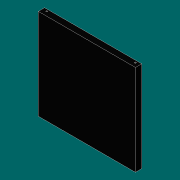
# Autodesk Inventor part: front
Saved by Autodesk Inventor 2016 SP1 (Build 200210100, 210)
## iProperties
Created: 2015-10-13
Part Number: front
Material: PC/ABS Plastic
Document SubType Name: Modeling
Designer: Sawaiz
Density: 0.357273 g/cm^3
Appearance: Smooth - Black
Author: Sawaiz
Autodesk Inventor part; units mm, degrees
ref_plane "YZ Plane" through (0, 0, 0) normal (1, 0, 0) x (0, 1, 0)
ref_plane "XZ Plane" through (0, 0, 0) normal (0, 1, 0) x (-1, 0, 0)
ref_plane "XY Plane" through (0, 0, 0) normal (0, 0, 1) x (1, 0, 0)
sketch "Sketch1" plane through (0, 0, 0) normal (1, 0, 0) x (0, 1, 0)
  line L0 (-73.025, -68.2625) -> (73.025, -68.2625)
  line L1 (73.025, -68.2625) -> (73.025, 68.2625)
  line L2 (73.025, 68.2625) -> (-73.025, 68.2625)
  line L3 (-73.025, 68.2625) -> (-73.025, -68.2625)
  line L4 (-73.025, -68.2625) -> (73.025, 68.2625) construction
  line L5 (73.025, -68.2625) -> (-73.025, 68.2625) construction
  point P0 (0, 0)
  dimension "d0" = 146.05
  dimension "d1" = 136.525
  constraints: 12 end point, 2 midpoint, 2 parallel, 1 horizontal, 1 perpendicular
  measures "d0" distance of L2.end L1.end
  measures "d1" distance of L1.end L0.end
extrude "Extrusion1" add sketch "Sketch1" along normal blind 9.525
sketch "Sketch5" plane through (0, -73.025, 68.2625) normal (0, 0, 1) x (1, 0, 0)
  line L0 (0, 146.05) -> (0, 0) projected
  line L1 (0, 0) -> (9.525, 0) projected
  line L2 (9.525, 146.05) -> (9.525, 0) projected
  line L3 (0, 146.05) -> (9.525, 146.05) projected
  line L4 (0, 146.05) -> (9.525, 146.05) projected
  line L5 (3.175, 146.05) -> (3.175, 0)
  point P0 (0, 73.025)
  point P1 (3.175, 139.7)
  point P2 (3.175, 6.35)
  dimension "d35" = 6.35
  dimension "d36" = 6.35
  dimension "d37" = 6.35
  constraints: 4 point on line, 2 end point, 1 parallel
  measures "d35" distance between parallel lines of L2 L5
  measures "d36" distance from line of L1 point (3.175, 6.35)
  measures "d37" distance from line of L3 point (3.175, 139.7)
hole "Hole3" at (3.175, 66.675, 68.2625) at (3.175, -66.675, 68.2625) direction (0, 0, -1) diameter 2.156 depth 8.865 tip angle 118 thread size "4-40 UNC" class "2B" standard "ANSI Unified Screw Threads"
equation "\"d0\" = width + 2 * frameAcrylicThickness"
equation "\"d1\" = height + 1.5 * internalAcrylicThickness"
equation "\"d2\" = frameAcrylicThickness"
equation "\"height\" = 127"
equation "\"width\" = 127"
equation "\"frameAcrylicThickness\" = 9.525"
equation "\"internalAcrylicThickness\" = 6.35"
equation "\"depth\" = 273.05"
equation "\"mirrorAngle\" = 5deg"
equation "\"detectorWidth\" = 52"
equation "\"detectorHeight\" = 52"
equation "\"mirrorThickness\" = 3.175"
equation "\"fresnelThickness\" = 0.1"
equation "\"focalLength\" = 76.2"
equation "\"ior\" = 1.49"
equation "\"centerThickness\" = 1.524"
equation "\"fresnelAngle\" = 90deg"
equation "\"fresnelEffectiveDiameter\" = 152.4"
equation "\"oRingWidth\" = 1.5875"
equation "\"sensorHolderDepth\" = 19.05"
equation "\"aerogelClearence\" = 3.175"
equation "\"backplaneHoleOffsett\" = 6.35"
equation "\"backplanePCBHeight\" = 76.2"
equation "\"backplanePCBWidth\" = 76.2"
equation "\"backplanePostionOffsett\" = 12.7"
equation "\"moduleSlotClearence\" = 0.79375"
body "Solid1"
